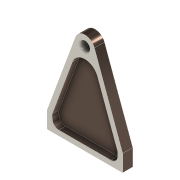
# Autodesk Inventor part: Bearing Short
Saved by Autodesk Inventor 2022.2 (Build 262287010, 287A)
## iProperties
Created: 2022-12-29
Part Number: Bearing Short
Material: Steel
Document SubType Name: Modeling
Designer: User
Mass: 63.2945 g
Surface Area: 67.9627 cm^2
Volume: 8.063 cm^3
Density: 7.85 g/cm^3
Appearance: Gunmetal - Antique Polished
Author: User
Autodesk Inventor part; units mm, degrees
ref_plane "YZ Plane" through (0, 0, 0) normal (1, 0, 0) x (0, 1, 0)
ref_plane "XZ Plane" through (0, 0, 0) normal (0, 1, 0) x (-1, 0, 0)
ref_plane "XY Plane" through (0, 0, 0) normal (0, 0, 1) x (1, 0, 0)
sketch "Sketch1" plane through (0, 0, 0) normal (0, 0, 1) x (1, 0, 0)
  line L0 (-22.5, 0) -> (22.5, 0)
  line L1 (22.5, 0) -> (22.5, 10)
  line L2 (22.5, 10) -> (5.6342, 56.0629)
  arc A0 (5.6342, 56.0629) -> (-5.6342, 56.0629) centre (0, 54) ccw
  line L3 (-5.6342, 56.0629) -> (-22.5, 10)
  line L4 (-22.5, 10) -> (-22.5, 0)
  point P0 (0, 0)
  point P1 (0, 0)
  dimension "d0" = 45
  dimension "d1" = 10
  dimension "d2" = 6
  dimension "d3" = 54
  constraints: 10 end point, 2 point on circle, 2 tangent, 1 centre point, 1 coincident, 1 equal length, 1 horizontal, 1 midpoint, 1 parallel, 1 perpendicular, 1 vertical alignment
  measures "d0" distance of L0.start L0.end
  measures "d1" distance of L3.end L0.start
  measures "d2" radius of A0
  measures "d3" distance from line of L0 A0.centre
extrude "Extrusion1" add sketch "Sketch1" along normal blind 6
sketch "Sketch2" plane through (0, 0, 6) normal (0, 0, 1) x (1, 0, 0)
  line L0 (22.5, 0) -> (22.5, 10) projected
  line L1 (22.5, 10) -> (5.6342, 56.0629) projected
  line L2 (-5.6342, 56.0629) -> (-22.5, 10) projected
  line L3 (-22.5, 10) -> (-22.5, 0) projected
  line L4 (-22.5, 0) -> (22.5, 0) projected
  line L5 (-19.5, 9.468) -> (-7.5123, 42.2083)
  line L6 (7.5123, 42.2083) -> (19.5, 9.468)
  line L7 (19.5, 9.468) -> (19.5, 7)
  line L8 (15.5, 3) -> (-15.5, 3)
  line L9 (-19.5, 7) -> (-19.5, 9.468)
  arc A0 (7.5123, 42.2083) -> (-7.5123, 42.2083) centre (0, 39.4577) ccw
  arc A1 (-19.5, 7) -> (-15.5, 3) centre (-15.5, 7) ccw
  arc A2 (15.5, 3) -> (19.5, 7) centre (15.5, 7) ccw
  point P0 (0, 0)
  dimension "d6" = 3
  dimension "d7" = 8
  dimension "d8" = 3
  dimension "d9" = 4
  constraints: 10 end point, 6 point on circle, 6 tangent, 3 centre point, 1 equal radius, 3 other
  measures "d6" distance between parallel lines of L2 L5
  measures "d7" radius of A0
  measures "d8" distance between parallel lines of L4 L8
  measures "d9" radius of A1
extrude "Extrusion2" cut sketch "Sketch2" against normal blind 4
sketch "Sketch3" plane through (0, 0, 6) normal (0, 0, 1) x (1, 0, 0)
  arc A0 (5.6342, 56.0629) -> (-5.6342, 56.0629) centre (0, 54) ccw projected
  point P0 (0, 0)
  constraints: 1 coincident
hole "Hole1" at (0, 54, 6) direction (0, 0, -1) diameter 6 end through all
body "Solid1"
